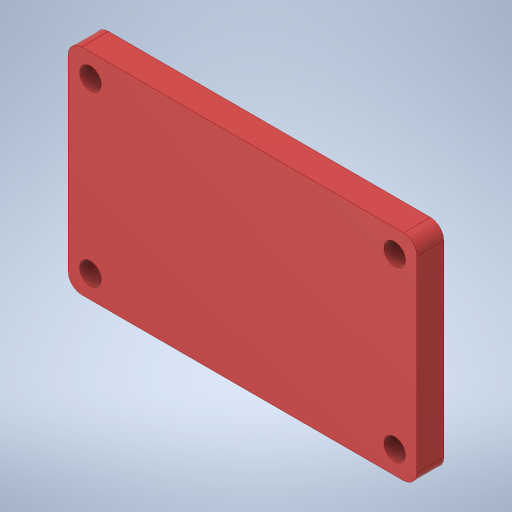
# Autodesk Inventor part: LL-001
Saved by Autodesk Inventor 2023.3 (Build 273359000, 359)
## iProperties
Created: 2024-01-25
Part Number: LL-001
Material: ABS Plastic
Document SubType Name: Modeling
Designer: mavericks
Density: 1.06 g/cm^3
Appearance: Smooth - Red
Author: mavericks
Autodesk Inventor part; units mm, degrees
ref_plane "YZ Plane" through (0, 0, 0) normal (1, 0, 0) x (0, 1, 0)
ref_plane "XZ Plane" through (0, 0, 0) normal (0, 1, 0) x (-1, 0, 0)
ref_plane "XY Plane" through (0, 0, 0) normal (0, 0, 1) x (1, 0, 0)
sketch "Sketch1" plane through (0, 0, 0) normal (0, 0, 1) x (1, 0, 0)
  line L0 (0, 0) -> (82.55, 0)
  line L1 (82.55, 0) -> (82.55, 50.8)
  line L2 (82.55, 50.8) -> (0, 50.8)
  line L3 (0, 50.8) -> (0, 0)
  dimension "d0" = 50.8
  dimension "d1" = 82.55
  constraints: 8 end point, 2 parallel, 1 horizontal, 1 perpendicular
  measures "d0" distance of L2.end L0.start
  measures "d1" distance of L0.start L0.end
extrude "Extrusion1" add sketch "Sketch1" along normal blind 6.35
fillet "Fillet1" radius 3.175 4 edges at (82.55, 50.8, 3.175) (82.55, 0, 3.175) (0, 0, 3.175) (0, 50.8, 3.175)
sketch "Sketch2" plane through (0, 0, 6.35) normal (0, 0, 1) x (1, 0, 0)
  line L0 (5.2705, 45.4025) -> (77.2795, 45.4025) construction
  line L1 (77.2795, 45.4025) -> (77.2795, 5.3975) construction
  line L2 (77.2795, 5.3975) -> (5.2705, 5.3975) construction
  line L3 (5.2705, 5.3975) -> (5.2705, 45.4025) construction
  line L4 (0, 47.625) -> (0, 3.175) construction
  line L5 (79.375, 50.8) -> (3.175, 50.8) construction
  point P0 (0, 0)
  point P1 (5.2705, 25.4)
  point P2 (0, 25.4)
  point P3 (41.275, 45.4025)
  point P4 (41.275, 50.8)
  dimension "d5" = 72.009
  dimension "d6" = 40.005
  constraints: 8 end point, 4 coincident, 4 midpoint, 2 parallel, 1 horizontal, 1 horizontal alignment, 1 perpendicular, 1 vertical alignment
  measures "d5" distance of L0.start L0.end
  measures "d6" distance of L2.end L0.start
hole "Hole1" at (5.2705, 45.4025, 6.35) at (77.2795, 45.4025, 6.35) at (77.2795, 5.3975, 6.35) at (5.2705, 5.3975, 6.35) direction (0, 0, -1) diameter 5.1054 end through all clearance for "Flat Head Machine Screw (82)" size "#10" standard "Ansi Unified Screw Threads"
body "Solid1"
